Autodesk Fusion 360 part; units mm, degrees
(part 2 of 6)
  line L1135 (-27.0711, 10) -> (-22.9289, 10)
  line L1136 (-22.9289, 10) -> (-20, 12.9289)
  line L1137 (-20, 12.9289) -> (-20, 17.0711)
  line L1138 (-20, 17.0711) -> (-22.9289, 20)
  line L1139 (-20, 17.0711) -> (-20, 12.9289)
  line L1140 (-17.0711, 20) -> (-20, 17.0711)
  line L1141 (-16.6569, 19) -> (-19, 16.6569)
  line L1142 (-13.3431, 19) -> (-16.6569, 19)
  line L1143 (-11, 16.6569) -> (-13.3431, 19)
  line L1144 (-11, 13.3431) -> (-11, 16.6569)
  line L1145 (-13.3431, 11) -> (-11, 13.3431)
  line L1146 (-16.6569, 11) -> (-13.3431, 11)
  line L1147 (-19, 13.3431) -> (-16.6569, 11)
  line L1148 (-19, 16.6569) -> (-19, 13.3431)
  line L1149 (-20, 12.9289) -> (-17.0711, 10)
  line L1150 (-17.0711, 10) -> (-12.9289, 10)
  line L1151 (-12.9289, 10) -> (-10, 12.9289)
  line L1152 (-10, 12.9289) -> (-10, 17.0711)
  line L1153 (-10, 17.0711) -> (-12.9289, 20)
  line L1154 (-10, 17.0711) -> (-10, 12.9289)
  line L1155 (-7.0711, 20) -> (-10, 17.0711)
  line L1156 (-6.6569, 19) -> (-9, 16.6569)
  line L1157 (-3.3431, 19) -> (-6.6569, 19)
  line L1158 (-1, 16.6569) -> (-3.3431, 19)
  line L1159 (-1, 13.3431) -> (-1, 16.6569)
  line L1160 (-3.3431, 11) -> (-1, 13.3431)
  line L1161 (-6.6569, 11) -> (-3.3431, 11)
  line L1162 (-9, 13.3431) -> (-6.6569, 11)
  line L1163 (-9, 16.6569) -> (-9, 13.3431)
  line L1164 (-10, 12.9289) -> (-7.0711, 10)
  line L1165 (-7.0711, 10) -> (-2.9289, 10)
  line L1166 (-2.9289, 10) -> (0, 12.9289)
  line L1167 (0, 12.9289) -> (0, 17.0711)
  line L1168 (0, 17.0711) -> (-2.9289, 20)
  line L1169 (0, 17.0711) -> (0, 12.9289)
  line L1170 (2.9289, 20) -> (0, 17.0711)
  line L1171 (3.3431, 19) -> (1, 16.6569)
  line L1172 (6.6569, 19) -> (3.3431, 19)
  line L1173 (9, 16.6569) -> (6.6569, 19)
  line L1174 (9, 13.3431) -> (9, 16.6569)
  line L1175 (6.6569, 11) -> (9, 13.3431)
  line L1176 (3.3431, 11) -> (6.6569, 11)
  line L1177 (1, 13.3431) -> (3.3431, 11)
  line L1178 (1, 16.6569) -> (1, 13.3431)
  line L1179 (0, 12.9289) -> (2.9289, 10)
  line L1180 (2.9289, 10) -> (7.0711, 10)
  line L1181 (7.0711, 10) -> (10, 12.9289)
  line L1182 (10, 12.9289) -> (10, 17.0711)
  line L1183 (10, 17.0711) -> (7.0711, 20)
  line L1184 (10, 17.0711) -> (10, 12.9289)
  line L1185 (12.9289, 20) -> (10, 17.0711)
  line L1186 (13.3431, 19) -> (11, 16.6569)
  line L1187 (16.6569, 19) -> (13.3431, 19)
  line L1188 (19, 16.6569) -> (16.6569, 19)
  line L1189 (19, 13.3431) -> (19, 16.6569)
  line L1190 (16.6569, 11) -> (19, 13.3431)
  line L1191 (13.3431, 11) -> (16.6569, 11)
  line L1192 (11, 13.3431) -> (13.3431, 11)
  line L1193 (11, 16.6569) -> (11, 13.3431)
  line L1194 (10, 12.9289) -> (12.9289, 10)
  line L1195 (12.9289, 10) -> (17.0711, 10)
  line L1196 (17.0711, 10) -> (20, 12.9289)
  line L1197 (20, 12.9289) -> (20, 17.0711)
  line L1198 (20, 17.0711) -> (17.0711, 20)
  line L1199 (20, 17.0711) -> (20, 12.9289)
  line L1200 (22.9289, 20) -> (20, 17.0711)
  line L1201 (23.3431, 19) -> (21, 16.6569)
  line L1202 (26.6569, 19) -> (23.3431, 19)
  line L1203 (29, 16.6569) -> (26.6569, 19)
  line L1204 (29, 13.3431) -> (29, 16.6569)
  line L1205 (26.6569, 11) -> (29, 13.3431)
  line L1206 (23.3431, 11) -> (26.6569, 11)
  line L1207 (21, 13.3431) -> (23.3431, 11)
  line L1208 (21, 16.6569) -> (21, 13.3431)
  line L1209 (20, 12.9289) -> (22.9289, 10)
  line L1210 (22.9289, 10) -> (27.0711, 10)
  line L1211 (27.0711, 10) -> (30, 12.9289)
  line L1212 (30, 12.9289) -> (30, 17.0711)
  line L1213 (30, 17.0711) -> (27.0711, 20)
  line L1214 (30, 17.0711) -> (30, 12.9289)
  line L1215 (32.9289, 20) -> (30, 17.0711)
  line L1216 (33.3431, 19) -> (31, 16.6569)
  line L1217 (36.6569, 19) -> (33.3431, 19)
  line L1218 (39, 16.6569) -> (36.6569, 19)
  line L1219 (39, 13.3431) -> (39, 16.6569)
  line L1220 (36.6569, 11) -> (39, 13.3431)
  line L1221 (33.3431, 11) -> (36.6569, 11)
  line L1222 (31, 13.3431) -> (33.3431, 11)
  line L1223 (31, 16.6569) -> (31, 13.3431)
  line L1224 (30, 12.9289) -> (32.9289, 10)
  line L1225 (32.9289, 10) -> (37.0711, 10)
  line L1226 (37.0711, 10) -> (40, 12.9289)
  line L1227 (40, 12.9289) -> (40, 17.0711)
  line L1228 (40, 17.0711) -> (37.0711, 20)
  line L1229 (40, 17.0711) -> (40, 12.9289)
  line L1230 (42.9289, 20) -> (40, 17.0711)
  line L1231 (43.3431, 19) -> (41, 16.6569)
  line L1232 (46.6569, 19) -> (43.3431, 19)
  line L1233 (49, 16.6569) -> (46.6569, 19)
  line L1234 (49, 13.3431) -> (49, 16.6569)
  line L1235 (46.6569, 11) -> (49, 13.3431)
  line L1236 (43.3431, 11) -> (46.6569, 11)
  line L1237 (41, 13.3431) -> (43.3431, 11)
  line L1238 (41, 16.6569) -> (41, 13.3431)
  line L1239 (40, 12.9289) -> (42.9289, 10)
  line L1240 (42.9289, 10) -> (47.0711, 10)
  line L1241 (47.0711, 10) -> (50, 12.9289)
  line L1242 (50, 12.9289) -> (50, 17.0711)
  line L1243 (50, 17.0711) -> (47.0711, 20)
  line L1244 (50, 17.0711) -> (50, 12.9289)
  line L1245 (52.9289, 20) -> (50, 17.0711)
  line L1246 (53.3431, 19) -> (51, 16.6569)
  line L1247 (56.6569, 19) -> (53.3431, 19)
  line L1248 (59, 16.6569) -> (56.6569, 19)
  line L1249 (59, 13.3431) -> (59, 16.6569)
  line L1250 (56.6569, 11) -> (59, 13.3431)
  line L1251 (53.3431, 11) -> (56.6569, 11)
  line L1252 (51, 13.3431) -> (53.3431, 11)
  line L1253 (51, 16.6569) -> (51, 13.3431)
  line L1254 (50, 12.9289) -> (52.9289, 10)
  line L1255 (52.9289, 10) -> (57.0711, 10)
  line L1256 (57.0711, 10) -> (60, 12.9289)
  line L1257 (60, 12.9289) -> (60, 17.0711)
  line L1258 (60, 17.0711) -> (57.0711, 20)
  line L1259 (60, 17.0711) -> (60, 12.9289)
  line L1260 (62.9289, 20) -> (60, 17.0711)
  line L1261 (63.3431, 19) -> (61, 16.6569)
  line L1262 (66.6569, 19) -> (63.3431, 19)
  line L1263 (69, 16.6569) -> (66.6569, 19)
  line L1264 (69, 13.3431) -> (69, 16.6569)
  line L1265 (66.6569, 11) -> (69, 13.3431)
  line L1266 (63.3431, 11) -> (66.6569, 11)
  line L1267 (61, 13.3431) -> (63.3431, 11)
  line L1268 (61, 16.6569) -> (61, 13.3431)
  line L1269 (60, 12.9289) -> (62.9289, 10)
  line L1270 (62.9289, 10) -> (67.0711, 10)
  line L1271 (67.0711, 10) -> (70, 12.9289)
  line L1272 (70, 12.9289) -> (70, 17.0711)
  line L1273 (70, 17.0711) -> (67.0711, 20)
  line L1274 (-70, 7.0711) -> (-70, 2.9289)
  line L1275 (-67.0711, 10) -> (-70, 7.0711)
  line L1276 (-66.6569, 9) -> (-69, 6.6569)
  line L1277 (-63.3431, 9) -> (-66.6569, 9)
  line L1278 (-61, 6.6569) -> (-63.3431, 9)
  line L1279 (-61, 3.3431) -> (-61, 6.6569)
  line L1280 (-63.3431, 1) -> (-61, 3.3431)
  line L1281 (-66.6569, 1) -> (-63.3431, 1)
  line L1282 (-69, 3.3431) -> (-66.6569, 1)
  line L1283 (-69, 6.6569) -> (-69, 3.3431)
  line L1284 (-70, 2.9289) -> (-67.0711, 0)
  line L1285 (-67.0711, 0) -> (-62.9289, 0)
  line L1286 (-62.9289, 0) -> (-60, 2.9289)
  line L1287 (-60, 2.9289) -> (-60, 7.0711)
  line L1288 (-60, 7.0711) -> (-62.9289, 10)
  line L1289 (-60, 7.0711) -> (-60, 2.9289)
  line L1290 (-57.0711, 10) -> (-60, 7.0711)
  line L1291 (-56.6569, 9) -> (-59, 6.6569)
  line L1292 (-53.3431, 9) -> (-56.6569, 9)
  line L1293 (-51, 6.6569) -> (-53.3431, 9)
  line L1294 (-51, 3.3431) -> (-51, 6.6569)
  line L1295 (-53.3431, 1) -> (-51, 3.3431)
  line L1296 (-56.6569, 1) -> (-53.3431, 1)
  line L1297 (-59, 3.3431) -> (-56.6569, 1)
  line L1298 (-59, 6.6569) -> (-59, 3.3431)
  line L1299 (-60, 2.9289) -> (-57.0711, 0)
  line L1300 (-57.0711, 0) -> (-52.9289, 0)
  line L1301 (-52.9289, 0) -> (-50, 2.9289)
  line L1302 (-50, 2.9289) -> (-50, 7.0711)
  line L1303 (-50, 7.0711) -> (-52.9289, 10)
  line L1304 (-50, 7.0711) -> (-50, 2.9289)
  line L1305 (-47.0711, 10) -> (-50, 7.0711)
  line L1306 (-46.6569, 9) -> (-49, 6.6569)
  line L1307 (-43.3431, 9) -> (-46.6569, 9)
  line L1308 (-41, 6.6569) -> (-43.3431, 9)
  line L1309 (-41, 3.3431) -> (-41, 6.6569)
  line L1310 (-43.3431, 1) -> (-41, 3.3431)
  line L1311 (-46.6569, 1) -> (-43.3431, 1)
  line L1312 (-49, 3.3431) -> (-46.6569, 1)
  line L1313 (-49, 6.6569) -> (-49, 3.3431)
  line L1314 (-50, 2.9289) -> (-47.0711, 0)
  line L1315 (-47.0711, 0) -> (-42.9289, 0)
  line L1316 (-42.9289, 0) -> (-40, 2.9289)
  line L1317 (-40, 2.9289) -> (-40, 7.0711)
  line L1318 (-40, 7.0711) -> (-42.9289, 10)
  line L1319 (-40, 7.0711) -> (-40, 2.9289)
  line L1320 (-37.0711, 10) -> (-40, 7.0711)
  line L1321 (-36.6569, 9) -> (-39, 6.6569)
  line L1322 (-33.3431, 9) -> (-36.6569, 9)
  line L1323 (-31, 6.6569) -> (-33.3431, 9)
  line L1324 (-31, 3.3431) -> (-31, 6.6569)
  line L1325 (-33.3431, 1) -> (-31, 3.3431)
  line L1326 (-36.6569, 1) -> (-33.3431, 1)
  line L1327 (-39, 3.3431) -> (-36.6569, 1)
  line L1328 (-39, 6.6569) -> (-39, 3.3431)
  line L1329 (-40, 2.9289) -> (-37.0711, 0)
  line L1330 (-37.0711, 0) -> (-32.9289, 0)
  line L1331 (-32.9289, 0) -> (-30, 2.9289)
  line L1332 (-30, 2.9289) -> (-30, 7.0711)
  line L1333 (-30, 7.0711) -> (-32.9289, 10)
  line L1334 (-30, 7.0711) -> (-30, 2.9289)
  line L1335 (-27.0711, 10) -> (-30, 7.0711)
  line L1336 (-26.6569, 9) -> (-29, 6.6569)
  line L1337 (-23.3431, 9) -> (-26.6569, 9)
  line L1338 (-21, 6.6569) -> (-23.3431, 9)
  line L1339 (-21, 3.3431) -> (-21, 6.6569)
  line L1340 (-23.3431, 1) -> (-21, 3.3431)
  line L1341 (-26.6569, 1) -> (-23.3431, 1)
  line L1342 (-29, 3.3431) -> (-26.6569, 1)
  line L1343 (-29, 6.6569) -> (-29, 3.3431)
  line L1344 (-30, 2.9289) -> (-27.0711, 0)
  line L1345 (-27.0711, 0) -> (-22.9289, 0)
  line L1346 (-22.9289, 0) -> (-20, 2.9289)
  line L1347 (-20, 2.9289) -> (-20, 7.0711)
  line L1348 (-20, 7.0711) -> (-22.9289, 10)
  line L1349 (-20, 7.0711) -> (-20, 2.9289)
  line L1350 (-17.0711, 10) -> (-20, 7.0711)
  line L1351 (-16.6569, 9) -> (-19, 6.6569)
  line L1352 (-13.3431, 9) -> (-16.6569, 9)
  line L1353 (-11, 6.6569) -> (-13.3431, 9)
  line L1354 (-11, 3.3431) -> (-11, 6.6569)
  line L1355 (-13.3431, 1) -> (-11, 3.3431)
  line L1356 (-16.6569, 1) -> (-13.3431, 1)
  line L1357 (-19, 3.3431) -> (-16.6569, 1)
  line L1358 (-19, 6.6569) -> (-19, 3.3431)
  line L1359 (-20, 2.9289) -> (-17.0711, 0)
  line L1360 (-17.0711, 0) -> (-12.9289, 0)
  line L1361 (-12.9289, 0) -> (-10, 2.9289)
  line L1362 (-10, 2.9289) -> (-10, 7.0711)
  line L1363 (-10, 7.0711) -> (-12.9289, 10)
  line L1364 (-10, 7.0711) -> (-10, 2.9289)
  line L1365 (-7.0711, 10) -> (-10, 7.0711)
  line L1366 (-6.6569, 9) -> (-9, 6.6569)
  line L1367 (-3.3431, 9) -> (-6.6569, 9)
  line L1368 (-1, 6.6569) -> (-3.3431, 9)
  line L1369 (-1, 3.3431) -> (-1, 6.6569)
  line L1370 (-3.3431, 1) -> (-1, 3.3431)
  line L1371 (-6.6569, 1) -> (-3.3431, 1)
  line L1372 (-9, 3.3431) -> (-6.6569, 1)
  line L1373 (-9, 6.6569) -> (-9, 3.3431)
  line L1374 (-10, 2.9289) -> (-7.0711, 0)
  line L1375 (-7.0711, 0) -> (-2.9289, 0)
  line L1376 (-2.9289, 0) -> (0, 2.9289)
  line L1377 (0, 2.9289) -> (0, 7.0711)
  line L1378 (0, 7.0711) -> (-2.9289, 10)
  line L1379 (0, 7.0711) -> (0, 2.9289)
  line L1380 (2.9289, 10) -> (0, 7.0711)
  line L1381 (3.3431, 9) -> (1, 6.6569)
  line L1382 (6.6569, 9) -> (3.3431, 9)
  line L1383 (9, 6.6569) -> (6.6569, 9)
  line L1384 (9, 3.3431) -> (9, 6.6569)
  line L1385 (6.6569, 1) -> (9, 3.3431)
  line L1386 (3.3431, 1) -> (6.6569, 1)
  line L1387 (1, 3.3431) -> (3.3431, 1)
  line L1388 (1, 6.6569) -> (1, 3.3431)
  line L1389 (0, 2.9289) -> (2.9289, 0)
  line L1390 (2.9289, 0) -> (7.0711, 0)
  line L1391 (7.0711, 0) -> (10, 2.9289)
  line L1392 (10, 2.9289) -> (10, 7.0711)
  line L1393 (10, 7.0711) -> (7.0711, 10)
  line L1394 (10, 7.0711) -> (10, 2.9289)
  line L1395 (12.9289, 10) -> (10, 7.0711)
  line L1396 (13.3431, 9) -> (11, 6.6569)
  line L1397 (16.6569, 9) -> (13.3431, 9)
  line L1398 (19, 6.6569) -> (16.6569, 9)
  line L1399 (19, 3.3431) -> (19, 6.6569)
  line L1400 (16.6569, 1) -> (19, 3.3431)
  line L1401 (13.3431, 1) -> (16.6569, 1)
  line L1402 (11, 3.3431) -> (13.3431, 1)
  line L1403 (11, 6.6569) -> (11, 3.3431)
  line L1404 (10, 2.9289) -> (12.9289, 0)
  line L1405 (12.9289, 0) -> (17.0711, 0)
  line L1406 (17.0711, 0) -> (20, 2.9289)
  line L1407 (20, 2.9289) -> (20, 7.0711)
  line L1408 (20, 7.0711) -> (17.0711, 10)
  line L1409 (20, 7.0711) -> (20, 2.9289)
  line L1410 (22.9289, 10) -> (20, 7.0711)
  line L1411 (23.3431, 9) -> (21, 6.6569)
  line L1412 (26.6569, 9) -> (23.3431, 9)
  line L1413 (29, 6.6569) -> (26.6569, 9)
  line L1414 (29, 3.3431) -> (29, 6.6569)
  line L1415 (26.6569, 1) -> (29, 3.3431)
  line L1416 (23.3431, 1) -> (26.6569, 1)
  line L1417 (21, 3.3431) -> (23.3431, 1)
  line L1418 (21, 6.6569) -> (21, 3.3431)
  line L1419 (20, 2.9289) -> (22.9289, 0)
  line L1420 (22.9289, 0) -> (27.0711, 0)
  line L1421 (27.0711, 0) -> (30, 2.9289)
  line L1422 (30, 2.9289) -> (30, 7.0711)
  line L1423 (30, 7.0711) -> (27.0711, 10)
  line L1424 (30, 7.0711) -> (30, 2.9289)
  line L1425 (32.9289, 10) -> (30, 7.0711)
  line L1426 (33.3431, 9) -> (31, 6.6569)
  line L1427 (36.6569, 9) -> (33.3431, 9)
  line L1428 (39, 6.6569) -> (36.6569, 9)
  line L1429 (39, 3.3431) -> (39, 6.6569)
  line L1430 (36.6569, 1) -> (39, 3.3431)
  line L1431 (33.3431, 1) -> (36.6569, 1)
  line L1432 (31, 3.3431) -> (33.3431, 1)
  line L1433 (31, 6.6569) -> (31, 3.3431)
  line L1434 (30, 2.9289) -> (32.9289, 0)
  line L1435 (32.9289, 0) -> (37.0711, 0)
  line L1436 (37.0711, 0) -> (40, 2.9289)
  line L1437 (40, 2.9289) -> (40, 7.0711)
  line L1438 (40, 7.0711) -> (37.0711, 10)
  line L1439 (40, 7.0711) -> (40, 2.9289)
  line L1440 (42.9289, 10) -> (40, 7.0711)
  line L1441 (43.3431, 9) -> (41, 6.6569)
  line L1442 (46.6569, 9) -> (43.3431, 9)
  line L1443 (49, 6.6569) -> (46.6569, 9)
  line L1444 (49, 3.3431) -> (49, 6.6569)
  line L1445 (46.6569, 1) -> (49, 3.3431)
  line L1446 (43.3431, 1) -> (46.6569, 1)
  line L1447 (41, 3.3431) -> (43.3431, 1)
  line L1448 (41, 6.6569) -> (41, 3.3431)
  line L1449 (40, 2.9289) -> (42.9289, 0)
  line L1450 (42.9289, 0) -> (47.0711, 0)
  line L1451 (47.0711, 0) -> (50, 2.9289)
  line L1452 (50, 2.9289) -> (50, 7.0711)
  line L1453 (50, 7.0711) -> (47.0711, 10)
  line L1454 (50, 7.0711) -> (50, 2.9289)
  line L1455 (52.9289, 10) -> (50, 7.0711)
  line L1456 (53.3431, 9) -> (51, 6.6569)
  line L1457 (56.6569, 9) -> (53.3431, 9)
  line L1458 (59, 6.6569) -> (56.6569, 9)
  line L1459 (59, 3.3431) -> (59, 6.6569)
  line L1460 (56.6569, 1) -> (59, 3.3431)
  line L1461 (53.3431, 1) -> (56.6569, 1)
  line L1462 (51, 3.3431) -> (53.3431, 1)
  line L1463 (51, 6.6569) -> (51, 3.3431)
  line L1464 (50, 2.9289) -> (52.9289, 0)
  line L1465 (52.9289, 0) -> (57.0711, 0)
  line L1466 (57.0711, 0) -> (60, 2.9289)
  line L1467 (60, 2.9289) -> (60, 7.0711)
  line L1468 (60, 7.0711) -> (57.0711, 10)
  line L1469 (60, 7.0711) -> (60, 2.9289)
  line L1470 (62.9289, 10) -> (60, 7.0711)
  line L1471 (63.3431, 9) -> (61, 6.6569)
  line L1472 (66.6569, 9) -> (63.3431, 9)
  line L1473 (69, 6.6569) -> (66.6569, 9)
  line L1474 (69, 3.3431) -> (69, 6.6569)
  line L1475 (66.6569, 1) -> (69, 3.3431)
  line L1476 (63.3431, 1) -> (66.6569, 1)
  line L1477 (61, 3.3431) -> (63.3431, 1)
  line L1478 (61, 6.6569) -> (61, 3.3431)
  line L1479 (60, 2.9289) -> (62.9289, 0)
  line L1480 (62.9289, 0) -> (67.0711, 0)
  line L1481 (67.0711, 0) -> (70, 2.9289)
  line L1482 (70, 2.9289) -> (70, 7.0711)
  line L1483 (70, 7.0711) -> (67.0711, 10)
  line L1484 (-70, -2.9289) -> (-70, -7.0711)
  line L1485 (-67.0711, 0) -> (-70, -2.9289)
  line L1486 (-66.6569, -1) -> (-69, -3.3431)
  line L1487 (-63.3431, -1) -> (-66.6569, -1)
  line L1488 (-61, -3.3431) -> (-63.3431, -1)
  line L1489 (-61, -6.6569) -> (-61, -3.3431)
  line L1490 (-63.3431, -9) -> (-61, -6.6569)
  line L1491 (-66.6569, -9) -> (-63.3431, -9)
  line L1492 (-69, -6.6569) -> (-66.6569, -9)
  line L1493 (-69, -3.3431) -> (-69, -6.6569)
  line L1494 (-70, -7.0711) -> (-67.0711, -10)
  line L1495 (-67.0711, -10) -> (-62.9289, -10)
  line L1496 (-62.9289, -10) -> (-60, -7.0711)
  line L1497 (-60, -7.0711) -> (-60, -2.9289)
  line L1498 (-60, -2.9289) -> (-62.9289, 0)
  line L1499 (-60, -2.9289) -> (-60, -7.0711)
  line L1500 (-57.0711, 0) -> (-60, -2.9289)
  line L1501 (-56.6569, -1) -> (-59, -3.3431)
  line L1502 (-53.3431, -1) -> (-56.6569, -1)
  line L1503 (-51, -3.3431) -> (-53.3431, -1)
  line L1504 (-51, -6.6569) -> (-51, -3.3431)
  line L1505 (-53.3431, -9) -> (-51, -6.6569)
  line L1506 (-56.6569, -9) -> (-53.3431, -9)
  line L1507 (-59, -6.6569) -> (-56.6569, -9)
  line L1508 (-59, -3.3431) -> (-59, -6.6569)
  line L1509 (-60, -7.0711) -> (-57.0711, -10)
  line L1510 (-57.0711, -10) -> (-52.9289, -10)
  line L1511 (-52.9289, -10) -> (-50, -7.0711)
  line L1512 (-50, -7.0711) -> (-50, -2.9289)
  line L1513 (-50, -2.9289) -> (-52.9289, 0)
  line L1514 (-50, -2.9289) -> (-50, -7.0711)
  line L1515 (-47.0711, 0) -> (-50, -2.9289)
  line L1516 (-46.6569, -1) -> (-49, -3.3431)
  line L1517 (-43.3431, -1) -> (-46.6569, -1)
  line L1518 (-41, -3.3431) -> (-43.3431, -1)
  line L1519 (-41, -6.6569) -> (-41, -3.3431)
  line L1520 (-43.3431, -9) -> (-41, -6.6569)
  line L1521 (-46.6569, -9) -> (-43.3431, -9)
  line L1522 (-49, -6.6569) -> (-46.6569, -9)
  line L1523 (-49, -3.3431) -> (-49, -6.6569)
  line L1524 (-50, -7.0711) -> (-47.0711, -10)
  line L1525 (-47.0711, -10) -> (-42.9289, -10)
  line L1526 (-42.9289, -10) -> (-40, -7.0711)
  line L1527 (-40, -7.0711) -> (-40, -2.9289)
  line L1528 (-40, -2.9289) -> (-42.9289, 0)
  line L1529 (-40, -2.9289) -> (-40, -7.0711)
  line L1530 (-37.0711, 0) -> (-40, -2.9289)
  line L1531 (-36.6569, -1) -> (-39, -3.3431)
  line L1532 (-33.3431, -1) -> (-36.6569, -1)
  line L1533 (-31, -3.3431) -> (-33.3431, -1)
  line L1534 (-31, -6.6569) -> (-31, -3.3431)
  line L1535 (-33.3431, -9) -> (-31, -6.6569)
  line L1536 (-36.6569, -9) -> (-33.3431, -9)
  line L1537 (-39, -6.6569) -> (-36.6569, -9)
  line L1538 (-39, -3.3431) -> (-39, -6.6569)
  line L1539 (-40, -7.0711) -> (-37.0711, -10)
  line L1540 (-37.0711, -10) -> (-32.9289, -10)
  line L1541 (-32.9289, -10) -> (-30, -7.0711)
  line L1542 (-30, -7.0711) -> (-30, -2.9289)
  line L1543 (-30, -2.9289) -> (-32.9289, 0)
  line L1544 (-30, -2.9289) -> (-30, -7.0711)
  line L1545 (-27.0711, 0) -> (-30, -2.9289)
  line L1546 (-26.6569, -1) -> (-29, -3.3431)
  line L1547 (-23.3431, -1) -> (-26.6569, -1)
  line L1548 (-21, -3.3431) -> (-23.3431, -1)
  line L1549 (-21, -6.6569) -> (-21, -3.3431)
  line L1550 (-23.3431, -9) -> (-21, -6.6569)
  line L1551 (-26.6569, -9) -> (-23.3431, -9)
  line L1552 (-29, -6.6569) -> (-26.6569, -9)
  line L1553 (-29, -3.3431) -> (-29, -6.6569)
  line L1554 (-30, -7.0711) -> (-27.0711, -10)
  line L1555 (-27.0711, -10) -> (-22.9289, -10)
  line L1556 (-22.9289, -10) -> (-20, -7.0711)
  line L1557 (-20, -7.0711) -> (-20, -2.9289)
  line L1558 (-20, -2.9289) -> (-22.9289, 0)
  line L1559 (-20, -2.9289) -> (-20, -7.0711)
  line L1560 (-17.0711, 0) -> (-20, -2.9289)
  line L1561 (-16.6569, -1) -> (-19, -3.3431)
  line L1562 (-13.3431, -1) -> (-16.6569, -1)
  line L1563 (-11, -3.3431) -> (-13.3431, -1)
  line L1564 (-11, -6.6569) -> (-11, -3.3431)
  line L1565 (-13.3431, -9) -> (-11, -6.6569)
  line L1566 (-16.6569, -9) -> (-13.3431, -9)
  line L1567 (-19, -6.6569) -> (-16.6569, -9)
  line L1568 (-19, -3.3431) -> (-19, -6.6569)
  line L1569 (-20, -7.0711) -> (-17.0711, -10)
  line L1570 (-17.0711, -10) -> (-12.9289, -10)
  line L1571 (-12.9289, -10) -> (-10, -7.0711)
  line L1572 (-10, -7.0711) -> (-10, -2.9289)
  line L1573 (-10, -2.9289) -> (-12.9289, 0)
  line L1574 (-10, -2.9289) -> (-10, -7.0711)
  line L1575 (-7.0711, 0) -> (-10, -2.9289)
  line L1576 (-6.6569, -1) -> (-9, -3.3431)
  line L1577 (-3.3431, -1) -> (-6.6569, -1)
  line L1578 (-1, -3.3431) -> (-3.3431, -1)
  line L1579 (-1, -6.6569) -> (-1, -3.3431)
  line L1580 (-3.3431, -9) -> (-1, -6.6569)
  line L1581 (-6.6569, -9) -> (-3.3431, -9)
  line L1582 (-9, -6.6569) -> (-6.6569, -9)
  line L1583 (-9, -3.3431) -> (-9, -6.6569)
  line L1584 (-10, -7.0711) -> (-7.0711, -10)
  line L1585 (-7.0711, -10) -> (-2.9289, -10)
  line L1586 (-2.9289, -10) -> (0, -7.0711)
  line L1587 (0, -7.0711) -> (0, -2.9289)
  line L1588 (0, -2.9289) -> (-2.9289, 0)
  line L1589 (0, -2.9289) -> (0, -7.0711)
  line L1590 (2.9289, 0) -> (0, -2.9289)
  line L1591 (3.3431, -1) -> (1, -3.3431)
  line L1592 (6.6569, -1) -> (3.3431, -1)
  line L1593 (9, -3.3431) -> (6.6569, -1)
  line L1594 (9, -6.6569) -> (9, -3.3431)
  line L1595 (6.6569, -9) -> (9, -6.6569)
  line L1596 (3.3431, -9) -> (6.6569, -9)
  line L1597 (1, -6.6569) -> (3.3431, -9)
  line L1598 (1, -3.3431) -> (1, -6.6569)
  line L1599 (0, -7.0711) -> (2.9289, -10)
  line L1600 (2.9289, -10) -> (7.0711, -10)
  line L1601 (7.0711, -10) -> (10, -7.0711)
  line L1602 (10, -7.0711) -> (10, -2.9289)
  line L1603 (10, -2.9289) -> (7.0711, 0)
  line L1604 (10, -2.9289) -> (10, -7.0711)
  line L1605 (12.9289, 0) -> (10, -2.9289)
  line L1606 (13.3431, -1) -> (11, -3.3431)
  line L1607 (16.6569, -1) -> (13.3431, -1)
  line L1608 (19, -3.3431) -> (16.6569, -1)
  line L1609 (19, -6.6569) -> (19, -3.3431)
  line L1610 (16.6569, -9) -> (19, -6.6569)
  line L1611 (13.3431, -9) -> (16.6569, -9)
  line L1612 (11, -6.6569) -> (13.3431, -9)
  line L1613 (11, -3.3431) -> (11, -6.6569)
  line L1614 (10, -7.0711) -> (12.9289, -10)
  line L1615 (12.9289, -10) -> (17.0711, -10)
  line L1616 (17.0711, -10) -> (20, -7.0711)
  line L1617 (20, -7.0711) -> (20, -2.9289)
  line L1618 (20, -2.9289) -> (17.0711, 0)
  line L1619 (20, -2.9289) -> (20, -7.0711)
  line L1620 (22.9289, 0) -> (20, -2.9289)
  line L1621 (23.3431, -1) -> (21, -3.3431)
  line L1622 (26.6569, -1) -> (23.3431, -1)
  line L1623 (29, -3.3431) -> (26.6569, -1)
  line L1624 (29, -6.6569) -> (29, -3.3431)
  line L1625 (26.6569, -9) -> (29, -6.6569)
  line L1626 (23.3431, -9) -> (26.6569, -9)
  line L1627 (21, -6.6569) -> (23.3431, -9)
  line L1628 (21, -3.3431) -> (21, -6.6569)
  line L1629 (20, -7.0711) -> (22.9289, -10)
  line L1630 (22.9289, -10) -> (27.0711, -10)
  line L1631 (27.0711, -10) -> (30, -7.0711)
  line L1632 (30, -7.0711) -> (30, -2.9289)
  line L1633 (30, -2.9289) -> (27.0711, 0)
  line L1634 (30, -2.9289) -> (30, -7.0711)
  line L1635 (32.9289, 0) -> (30, -2.9289)
  line L1636 (33.3431, -1) -> (31, -3.3431)
  line L1637 (36.6569, -1) -> (33.3431, -1)
  line L1638 (39, -3.3431) -> (36.6569, -1)
  line L1639 (39, -6.6569) -> (39, -3.3431)
  line L1640 (36.6569, -9) -> (39, -6.6569)
  line L1641 (33.3431, -9) -> (36.6569, -9)
  line L1642 (31, -6.6569) -> (33.3431, -9)
  line L1643 (31, -3.3431) -> (31, -6.6569)
  line L1644 (30, -7.0711) -> (32.9289, -10)
  line L1645 (32.9289, -10) -> (37.0711, -10)
  line L1646 (37.0711, -10) -> (40, -7.0711)
  line L1647 (40, -7.0711) -> (40, -2.9289)
  line L1648 (40, -2.9289) -> (37.0711, 0)
  line L1649 (40, -2.9289) -> (40, -7.0711)
  line L1650 (42.9289, 0) -> (40, -2.9289)
  line L1651 (43.3431, -1) -> (41, -3.3431)
  line L1652 (46.6569, -1) -> (43.3431, -1)
  line L1653 (49, -3.3431) -> (46.6569, -1)
  line L1654 (49, -6.6569) -> (49, -3.3431)
  line L1655 (46.6569, -9) -> (49, -6.6569)
  line L1656 (43.3431, -9) -> (46.6569, -9)
  line L1657 (41, -6.6569) -> (43.3431, -9)
  line L1658 (41, -3.3431) -> (41, -6.6569)
  line L1659 (40, -7.0711) -> (42.9289, -10)
  line L1660 (42.9289, -10) -> (47.0711, -10)
  line L1661 (47.0711, -10) -> (50, -7.0711)
  line L1662 (50, -7.0711) -> (50, -2.9289)
  line L1663 (50, -2.9289) -> (47.0711, 0)
  line L1664 (50, -2.9289) -> (50, -7.0711)
  line L1665 (52.9289, 0) -> (50, -2.9289)
  line L1666 (53.3431, -1) -> (51, -3.3431)
  line L1667 (56.6569, -1) -> (53.3431, -1)
  line L1668 (59, -3.3431) -> (56.6569, -1)
  line L1669 (59, -6.6569) -> (59, -3.3431)
  line L1670 (56.6569, -9) -> (59, -6.6569)
  line L1671 (53.3431, -9) -> (56.6569, -9)
  line L1672 (51, -6.6569) -> (53.3431, -9)
  line L1673 (51, -3.3431) -> (51, -6.6569)
  line L1674 (50, -7.0711) -> (52.9289, -10)
  line L1675 (52.9289, -10) -> (57.0711, -10)
  line L1676 (57.0711, -10) -> (60, -7.0711)
  line L1677 (60, -7.0711) -> (60, -2.9289)
  line L1678 (60, -2.9289) -> (57.0711, 0)
  line L1679 (60, -2.9289) -> (60, -7.0711)
  line L1680 (62.9289, 0) -> (60, -2.9289)
  line L1681 (63.3431, -1) -> (61, -3.3431)
  line L1682 (66.6569, -1) -> (63.3431, -1)
  line L1683 (69, -3.3431) -> (66.6569, -1)
  line L1684 (69, -6.6569) -> (69, -3.3431)
  line L1685 (66.6569, -9) -> (69, -6.6569)
  line L1686 (63.3431, -9) -> (66.6569, -9)
  line L1687 (61, -6.6569) -> (63.3431, -9)
  line L1688 (61, -3.3431) -> (61, -6.6569)
  line L1689 (60, -7.0711) -> (62.9289, -10)
  line L1690 (62.9289, -10) -> (67.0711, -10)
  line L1691 (67.0711, -10) -> (70, -7.0711)
  line L1692 (70, -7.0711) -> (70, -2.9289)
  line L1693 (70, -2.9289) -> (67.0711, 0)
  line L1694 (-70, -12.9289) -> (-70, -17.0711)
  line L1695 (-67.0711, -10) -> (-70, -12.9289)
  line L1696 (-66.6569, -11) -> (-69, -13.3431)
  line L1697 (-63.3431, -11) -> (-66.6569, -11)
  line L1698 (-61, -13.3431) -> (-63.3431, -11)
  line L1699 (-61, -16.6569) -> (-61, -13.3431)
  line L1700 (-63.3431, -19) -> (-61, -16.6569)
  line L1701 (-66.6569, -19) -> (-63.3431, -19)
  line L1702 (-69, -16.6569) -> (-66.6569, -19)
  line L1703 (-69, -13.3431) -> (-69, -16.6569)
  line L1704 (-70, -17.0711) -> (-67.0711, -20)
  line L1705 (-67.0711, -20) -> (-62.9289, -20)
  line L1706 (-62.9289, -20) -> (-60, -17.0711)
  line L1707 (-60, -17.0711) -> (-60, -12.9289)
  line L1708 (-60, -12.9289) -> (-62.9289, -10)
  line L1709 (-60, -12.9289) -> (-60, -17.0711)
  line L1710 (-57.0711, -10) -> (-60, -12.9289)
  line L1711 (-56.6569, -11) -> (-59, -13.3431)
  line L1712 (-53.3431, -11) -> (-56.6569, -11)
  line L1713 (-51, -13.3431) -> (-53.3431, -11)
  line L1714 (-51, -16.6569) -> (-51, -13.3431)
  line L1715 (-53.3431, -19) -> (-51, -16.6569)
  line L1716 (-56.6569, -19) -> (-53.3431, -19)
  line L1717 (-59, -16.6569) -> (-56.6569, -19)
  line L1718 (-59, -13.3431) -> (-59, -16.6569)
  line L1719 (-60, -17.0711) -> (-57.0711, -20)
  line L1720 (-57.0711, -20) -> (-52.9289, -20)
  line L1721 (-52.9289, -20) -> (-50, -17.0711)
  line L1722 (-50, -17.0711) -> (-50, -12.9289)
  line L1723 (-50, -12.9289) -> (-52.9289, -10)
  line L1724 (-50, -12.9289) -> (-50, -17.0711)
  line L1725 (-47.0711, -10) -> (-50, -12.9289)
  line L1726 (-46.6569, -11) -> (-49, -13.3431)
  line L1727 (-43.3431, -11) -> (-46.6569, -11)
  line L1728 (-41, -13.3431) -> (-43.3431, -11)
  line L1729 (-41, -16.6569) -> (-41, -13.3431)
  line L1730 (-43.3431, -19) -> (-41, -16.6569)
  line L1731 (-46.6569, -19) -> (-43.3431, -19)
  line L1732 (-49, -16.6569) -> (-46.6569, -19)
  line L1733 (-49, -13.3431) -> (-49, -16.6569)
  line L1734 (-50, -17.0711) -> (-47.0711, -20)
  line L1735 (-47.0711, -20) -> (-42.9289, -20)
  line L1736 (-42.9289, -20) -> (-40, -17.0711)
  line L1737 (-40, -17.0711) -> (-40, -12.9289)
  line L1738 (-40, -12.9289) -> (-42.9289, -10)
  line L1739 (-40, -12.9289) -> (-40, -17.0711)
  line L1740 (-37.0711, -10) -> (-40, -12.9289)
  line L1741 (-36.6569, -11) -> (-39, -13.3431)
  line L1742 (-33.3431, -11) -> (-36.6569, -11)
  line L1743 (-31, -13.3431) -> (-33.3431, -11)
  line L1744 (-31, -16.6569) -> (-31, -13.3431)
  line L1745 (-33.3431, -19) -> (-31, -16.6569)
  line L1746 (-36.6569, -19) -> (-33.3431, -19)
  line L1747 (-39, -16.6569) -> (-36.6569, -19)
  line L1748 (-39, -13.3431) -> (-39, -16.6569)
  line L1749 (-40, -17.0711) -> (-37.0711, -20)
  line L1750 (-37.0711, -20) -> (-32.9289, -20)
  line L1751 (-32.9289, -20) -> (-30, -17.0711)
  line L1752 (-30, -17.0711) -> (-30, -12.9289)
  line L1753 (-30, -12.9289) -> (-32.9289, -10)
  line L1754 (-30, -12.9289) -> (-30, -17.0711)
  line L1755 (-27.0711, -10) -> (-30, -12.9289)
  line L1756 (-26.6569, -11) -> (-29, -13.3431)
  line L1757 (-23.3431, -11) -> (-26.6569, -11)
  line L1758 (-21, -13.3431) -> (-23.3431, -11)
  line L1759 (-21, -16.6569) -> (-21, -13.3431)
  line L1760 (-23.3431, -19) -> (-21, -16.6569)
  line L1761 (-26.6569, -19) -> (-23.3431, -19)
  line L1762 (-29, -16.6569) -> (-26.6569, -19)
  line L1763 (-29, -13.3431) -> (-29, -16.6569)
  line L1764 (-30, -17.0711) -> (-27.0711, -20)
  line L1765 (-27.0711, -20) -> (-22.9289, -20)
  line L1766 (-22.9289, -20) -> (-20, -17.0711)
  line L1767 (-20, -17.0711) -> (-20, -12.9289)
  line L1768 (-20, -12.9289) -> (-22.9289, -10)
  line L1769 (-20, -12.9289) -> (-20, -17.0711)
  line L1770 (-17.0711, -10) -> (-20, -12.9289)
  line L1771 (-16.6569, -11) -> (-19, -13.3431)
  line L1772 (-13.3431, -11) -> (-16.6569, -11)
  line L1773 (-11, -13.3431) -> (-13.3431, -11)
  line L1774 (-11, -16.6569) -> (-11, -13.3431)
  line L1775 (-13.3431, -19) -> (-11, -16.6569)
  line L1776 (-16.6569, -19) -> (-13.3431, -19)
  line L1777 (-19, -16.6569) -> (-16.6569, -19)
  line L1778 (-19, -13.3431) -> (-19, -16.6569)
  line L1779 (-20, -17.0711) -> (-17.0711, -20)
  line L1780 (-17.0711, -20) -> (-12.9289, -20)
  line L1781 (-12.9289, -20) -> (-10, -17.0711)
  line L1782 (-10, -17.0711) -> (-10, -12.9289)
  line L1783 (-10, -12.9289) -> (-12.9289, -10)
  line L1784 (-10, -12.9289) -> (-10, -17.0711)
  line L1785 (-7.0711, -10) -> (-10, -12.9289)
  line L1786 (-6.6569, -11) -> (-9, -13.3431)
  line L1787 (-3.3431, -11) -> (-6.6569, -11)
  line L1788 (-1, -13.3431) -> (-3.3431, -11)
  line L1789 (-1, -16.6569) -> (-1, -13.3431)
  line L1790 (-3.3431, -19) -> (-1, -16.6569)
  line L1791 (-6.6569, -19) -> (-3.3431, -19)
  line L1792 (-9, -16.6569) -> (-6.6569, -19)
  line L1793 (-9, -13.3431) -> (-9, -16.6569)
  line L1794 (-10, -17.0711) -> (-7.0711, -20)
  line L1795 (-7.0711, -20) -> (-2.9289, -20)
  line L1796 (-2.9289, -20) -> (0, -17.0711)
  line L1797 (0, -17.0711) -> (0, -12.9289)
  line L1798 (0, -12.9289) -> (-2.9289, -10)
  line L1799 (0, -12.9289) -> (0, -17.0711)
  line L1800 (2.9289, -10) -> (0, -12.9289)
  line L1801 (3.3431, -11) -> (1, -13.3431)
  line L1802 (6.6569, -11) -> (3.3431, -11)
  line L1803 (9, -13.3431) -> (6.6569, -11)
  line L1804 (9, -16.6569) -> (9, -13.3431)
  line L1805 (6.6569, -19) -> (9, -16.6569)
  line L1806 (3.3431, -19) -> (6.6569, -19)
  line L1807 (1, -16.6569) -> (3.3431, -19)
  line L1808 (1, -13.3431) -> (1, -16.6569)
  line L1809 (0, -17.0711) -> (2.9289, -20)
  line L1810 (2.9289, -20) -> (7.0711, -20)
  line L1811 (7.0711, -20) -> (10, -17.0711)
  line L1812 (10, -17.0711) -> (10, -12.9289)
  line L1813 (10, -12.9289) -> (7.0711, -10)
  line L1814 (10, -12.9289) -> (10, -17.0711)
  line L1815 (12.9289, -10) -> (10, -12.9289)
  line L1816 (13.3431, -11) -> (11, -13.3431)
  line L1817 (16.6569, -11) -> (13.3431, -11)
  line L1818 (19, -13.3431) -> (16.6569, -11)
  line L1819 (19, -16.6569) -> (19, -13.3431)
  line L1820 (16.6569, -19) -> (19, -16.6569)
  line L1821 (13.3431, -19) -> (16.6569, -19)
  line L1822 (11, -16.6569) -> (13.3431, -19)
  line L1823 (11, -13.3431) -> (11, -16.6569)
  line L1824 (10, -17.0711) -> (12.9289, -20)
  line L1825 (12.9289, -20) -> (17.0711, -20)
  line L1826 (17.0711, -20) -> (20, -17.0711)
  line L1827 (20, -17.0711) -> (20, -12.9289)
  line L1828 (20, -12.9289) -> (17.0711, -10)
  line L1829 (20, -12.9289) -> (20, -17.0711)
  line L1830 (22.9289, -10) -> (20, -12.9289)
  line L1831 (23.3431, -11) -> (21, -13.3431)
  line L1832 (26.6569, -11) -> (23.3431, -11)
  line L1833 (29, -13.3431) -> (26.6569, -11)
  line L1834 (29, -16.6569) -> (29, -13.3431)
  line L1835 (26.6569, -19) -> (29, -16.6569)
  line L1836 (23.3431, -19) -> (26.6569, -19)
  line L1837 (21, -16.6569) -> (23.3431, -19)
  line L1838 (21, -13.3431) -> (21, -16.6569)
  line L1839 (20, -17.0711) -> (22.9289, -20)
  line L1840 (22.9289, -20) -> (27.0711, -20)
  line L1841 (27.0711, -20) -> (30, -17.0711)
  line L1842 (30, -17.0711) -> (30, -12.9289)
  line L1843 (30, -12.9289) -> (27.0711, -10)
  line L1844 (30, -12.9289) -> (30, -17.0711)
  line L1845 (32.9289, -10) -> (30, -12.9289)
  line L1846 (33.3431, -11) -> (31, -13.3431)
  line L1847 (36.6569, -11) -> (33.3431, -11)
  line L1848 (39, -13.3431) -> (36.6569, -11)
  line L1849 (39, -16.6569) -> (39, -13.3431)
  line L1850 (36.6569, -19) -> (39, -16.6569)
  line L1851 (33.3431, -19) -> (36.6569, -19)
  line L1852 (31, -16.6569) -> (33.3431, -19)
  line L1853 (31, -13.3431) -> (31, -16.6569)
  line L1854 (30, -17.0711) -> (32.9289, -20)
  line L1855 (32.9289, -20) -> (37.0711, -20)
  line L1856 (37.0711, -20) -> (40, -17.0711)
  line L1857 (40, -17.0711) -> (40, -12.9289)
  line L1858 (40, -12.9289) -> (37.0711, -10)
  line L1859 (40, -12.9289) -> (40, -17.0711)
  line L1860 (42.9289, -10) -> (40, -12.9289)
  line L1861 (43.3431, -11) -> (41, -13.3431)
  line L1862 (46.6569, -11) -> (43.3431, -11)
  line L1863 (49, -13.3431) -> (46.6569, -11)
  line L1864 (49, -16.6569) -> (49, -13.3431)
  line L1865 (46.6569, -19) -> (49, -16.6569)
  line L1866 (43.3431, -19) -> (46.6569, -19)
  line L1867 (41, -16.6569) -> (43.3431, -19)
  line L1868 (41, -13.3431) -> (41, -16.6569)
  line L1869 (40, -17.0711) -> (42.9289, -20)
  line L1870 (42.9289, -20) -> (47.0711, -20)
  line L1871 (47.0711, -20) -> (50, -17.0711)
  line L1872 (50, -17.0711) -> (50, -12.9289)
  line L1873 (50, -12.9289) -> (47.0711, -10)
  line L1874 (50, -12.9289) -> (50, -17.0711)
  line L1875 (52.9289, -10) -> (50, -12.9289)
  line L1876 (53.3431, -11) -> (51, -13.3431)
  line L1877 (56.6569, -11) -> (53.3431, -11)
  line L1878 (59, -13.3431) -> (56.6569, -11)
  line L1879 (59, -16.6569) -> (59, -13.3431)
  line L1880 (56.6569, -19) -> (59, -16.6569)
  line L1881 (53.3431, -19) -> (56.6569, -19)
  line L1882 (51, -16.6569) -> (53.3431, -19)
  line L1883 (51, -13.3431) -> (51, -16.6569)
  line L1884 (50, -17.0711) -> (52.9289, -20)
  line L1885 (52.9289, -20) -> (57.0711, -20)
  line L1886 (57.0711, -20) -> (60, -17.0711)
  line L1887 (60, -17.0711) -> (60, -12.9289)
  line L1888 (60, -12.9289) -> (57.0711, -10)
  line L1889 (60, -12.9289) -> (60, -17.0711)
  line L1890 (62.9289, -10) -> (60, -12.9289)
  line L1891 (63.3431, -11) -> (61, -13.3431)
  line L1892 (66.6569, -11) -> (63.3431, -11)
  line L1893 (69, -13.3431) -> (66.6569, -11)
  line L1894 (69, -16.6569) -> (69, -13.3431)
  line L1895 (66.6569, -19) -> (69, -16.6569)
  line L1896 (63.3431, -19) -> (66.6569, -19)
  line L1897 (61, -16.6569) -> (63.3431, -19)
  line L1898 (61, -13.3431) -> (61, -16.6569)
  line L1899 (60, -17.0711) -> (62.9289, -20)
  line L1900 (62.9289, -20) -> (67.0711, -20)
  line L1901 (67.0711, -20) -> (70, -17.0711)
  line L1902 (70, -17.0711) -> (70, -12.9289)
  line L1903 (70, -12.9289) -> (67.0711, -10)
  line L1904 (-70, -22.9289) -> (-70, -27.0711)
  line L1905 (-67.0711, -20) -> (-70, -22.9289)
  line L1906 (-66.6569, -21) -> (-69, -23.3431)
  line L1907 (-63.3431, -21) -> (-66.6569, -21)
  line L1908 (-61, -23.3431) -> (-63.3431, -21)
  line L1909 (-61, -26.6569) -> (-61, -23.3431)
  line L1910 (-63.3431, -29) -> (-61, -26.6569)
  line L1911 (-66.6569, -29) -> (-63.3431, -29)
  line L1912 (-69, -26.6569) -> (-66.6569, -29)
  line L1913 (-69, -23.3431) -> (-69, -26.6569)
  line L1914 (-70, -27.0711) -> (-67.0711, -30)
  line L1915 (-67.0711, -30) -> (-62.9289, -30)
  line L1916 (-62.9289, -30) -> (-60, -27.0711)
  line L1917 (-60, -27.0711) -> (-60, -22.9289)
  line L1918 (-60, -22.9289) -> (-62.9289, -20)
  line L1919 (-60, -22.9289) -> (-60, -27.0711)
  line L1920 (-57.0711, -20) -> (-60, -22.9289)
  line L1921 (-56.6569, -21) -> (-59, -23.3431)
  line L1922 (-53.3431, -21) -> (-56.6569, -21)
  line L1923 (-51, -23.3431) -> (-53.3431, -21)
  line L1924 (-51, -26.6569) -> (-51, -23.3431)
  line L1925 (-53.3431, -29) -> (-51, -26.6569)
  line L1926 (-56.6569, -29) -> (-53.3431, -29)
  line L1927 (-59, -26.6569) -> (-56.6569, -29)
  line L1928 (-59, -23.3431) -> (-59, -26.6569)
  line L1929 (-60, -27.0711) -> (-57.0711, -30)
  line L1930 (-57.0711, -30) -> (-52.9289, -30)
  line L1931 (-52.9289, -30) -> (-50, -27.0711)
  line L1932 (-50, -27.0711) -> (-50, -22.9289)
  line L1933 (-50, -22.9289) -> (-52.9289, -20)
  line L1934 (-50, -22.9289) -> (-50, -27.0711)
  line L1935 (-47.0711, -20) -> (-50, -22.9289)
  line L1936 (-46.6569, -21) -> (-49, -23.3431)
  line L1937 (-43.3431, -21) -> (-46.6569, -21)
  line L1938 (-41, -23.3431) -> (-43.3431, -21)
  line L1939 (-41, -26.6569) -> (-41, -23.3431)
  line L1940 (-43.3431, -29) -> (-41, -26.6569)
  line L1941 (-46.6569, -29) -> (-43.3431, -29)
  line L1942 (-49, -26.6569) -> (-46.6569, -29)
  line L1943 (-49, -23.3431) -> (-49, -26.6569)
  line L1944 (-50, -27.0711) -> (-47.0711, -30)
  line L1945 (-47.0711, -30) -> (-42.9289, -30)
  line L1946 (-42.9289, -30) -> (-40, -27.0711)
  line L1947 (-40, -27.0711) -> (-40, -22.9289)
  line L1948 (-40, -22.9289) -> (-42.9289, -20)
  line L1949 (-40, -22.9289) -> (-40, -27.0711)
  line L1950 (-37.0711, -20) -> (-40, -22.9289)
  line L1951 (-36.6569, -21) -> (-39, -23.3431)
  line L1952 (-33.3431, -21) -> (-36.6569, -21)
  line L1953 (-31, -23.3431) -> (-33.3431, -21)
  line L1954 (-31, -26.6569) -> (-31, -23.3431)
  line L1955 (-33.3431, -29) -> (-31, -26.6569)
  line L1956 (-36.6569, -29) -> (-33.3431, -29)
  line L1957 (-39, -26.6569) -> (-36.6569, -29)
  line L1958 (-39, -23.3431) -> (-39, -26.6569)
  line L1959 (-40, -27.0711) -> (-37.0711, -30)
  line L1960 (-37.0711, -30) -> (-32.9289, -30)
  line L1961 (-32.9289, -30) -> (-30, -27.0711)
  line L1962 (-30, -27.0711) -> (-30, -22.9289)
  line L1963 (-30, -22.9289) -> (-32.9289, -20)
  line L1964 (-30, -22.9289) -> (-30, -27.0711)
  line L1965 (-27.0711, -20) -> (-30, -22.9289)
  line L1966 (-26.6569, -21) -> (-29, -23.3431)
  line L1967 (-23.3431, -21) -> (-26.6569, -21)
  line L1968 (-21, -23.3431) -> (-23.3431, -21)
  line L1969 (-21, -26.6569) -> (-21, -23.3431)
  line L1970 (-23.3431, -29) -> (-21, -26.6569)
  line L1971 (-26.6569, -29) -> (-23.3431, -29)
  line L1972 (-29, -26.6569) -> (-26.6569, -29)
  line L1973 (-29, -23.3431) -> (-29, -26.6569)
  line L1974 (-30, -27.0711) -> (-27.0711, -30)
  line L1975 (-27.0711, -30) -> (-22.9289, -30)
  line L1976 (-22.9289, -30) -> (-20, -27.0711)
  line L1977 (-20, -27.0711) -> (-20, -22.9289)
  line L1978 (-20, -22.9289) -> (-22.9289, -20)
  line L1979 (-20, -22.9289) -> (-20, -27.0711)
  line L1980 (-17.0711, -20) -> (-20, -22.9289)
  line L1981 (-16.6569, -21) -> (-19, -23.3431)
  line L1982 (-13.3431, -21) -> (-16.6569, -21)
  line L1983 (-11, -23.3431) -> (-13.3431, -21)
  line L1984 (-11, -26.6569) -> (-11, -23.3431)
  line L1985 (-13.3431, -29) -> (-11, -26.6569)
  line L1986 (-16.6569, -29) -> (-13.3431, -29)
  line L1987 (-19, -26.6569) -> (-16.6569, -29)
  line L1988 (-19, -23.3431) -> (-19, -26.6569)
  line L1989 (-20, -27.0711) -> (-17.0711, -30)
  line L1990 (-17.0711, -30) -> (-12.9289, -30)
  line L1991 (-12.9289, -30) -> (-10, -27.0711)
  line L1992 (-10, -27.0711) -> (-10, -22.9289)
  line L1993 (-10, -22.9289) -> (-12.9289, -20)
  line L1994 (-10, -22.9289) -> (-10, -27.0711)
  line L1995 (-7.0711, -20) -> (-10, -22.9289)
  line L1996 (-6.6569, -21) -> (-9, -23.3431)
  line L1997 (-3.3431, -21) -> (-6.6569, -21)
  line L1998 (-1, -23.3431) -> (-3.3431, -21)
  line L1999 (-1, -26.6569) -> (-1, -23.3431)
  line L2000 (-3.3431, -29) -> (-1, -26.6569)
  line L2001 (-6.6569, -29) -> (-3.3431, -29)
  line L2002 (-9, -26.6569) -> (-6.6569, -29)
  line L2003 (-9, -23.3431) -> (-9, -26.6569)
  line L2004 (-10, -27.0711) -> (-7.0711, -30)
  line L2005 (-7.0711, -30) -> (-2.9289, -30)
  line L2006 (-2.9289, -30) -> (0, -27.0711)
  line L2007 (0, -27.0711) -> (0, -22.9289)
  line L2008 (0, -22.9289) -> (-2.9289, -20)
  line L2009 (0, -22.9289) -> (0, -27.0711)
  line L2010 (2.9289, -20) -> (0, -22.9289)
  line L2011 (3.3431, -21) -> (1, -23.3431)
  line L2012 (6.6569, -21) -> (3.3431, -21)
  line L2013 (9, -23.3431) -> (6.6569, -21)
  line L2014 (9, -26.6569) -> (9, -23.3431)
  line L2015 (6.6569, -29) -> (9, -26.6569)
  line L2016 (3.3431, -29) -> (6.6569, -29)
  line L2017 (1, -26.6569) -> (3.3431, -29)
  line L2018 (1, -23.3431) -> (1, -26.6569)
  line L2019 (0, -27.0711) -> (2.9289, -30)
  line L2020 (2.9289, -30) -> (7.0711, -30)
  line L2021 (7.0711, -30) -> (10, -27.0711)
  line L2022 (10, -27.0711) -> (10, -22.9289)
  line L2023 (10, -22.9289) -> (7.0711, -20)
  line L2024 (10, -22.9289) -> (10, -27.0711)
  line L2025 (12.9289, -20) -> (10, -22.9289)
  line L2026 (13.3431, -21) -> (11, -23.3431)
  line L2027 (16.6569, -21) -> (13.3431, -21)
  line L2028 (19, -23.3431) -> (16.6569, -21)
  line L2029 (19, -26.6569) -> (19, -23.3431)
  line L2030 (16.6569, -29) -> (19, -26.6569)
  line L2031 (13.3431, -29) -> (16.6569, -29)
  line L2032 (11, -26.6569) -> (13.3431, -29)
  line L2033 (11, -23.3431) -> (11, -26.6569)
  line L2034 (10, -27.0711) -> (12.9289, -30)
  line L2035 (12.9289, -30) -> (17.0711, -30)
  line L2036 (17.0711, -30) -> (20, -27.0711)
  line L2037 (20, -27.0711) -> (20, -22.9289)
  line L2038 (20, -22.9289) -> (17.0711, -20)
  line L2039 (20, -22.9289) -> (20, -27.0711)
  line L2040 (22.9289, -20) -> (20, -22.9289)
  line L2041 (23.3431, -21) -> (21, -23.3431)
  line L2042 (26.6569, -21) -> (23.3431, -21)
  line L2043 (29, -23.3431) -> (26.6569, -21)
  line L2044 (29, -26.6569) -> (29, -23.3431)
  line L2045 (26.6569, -29) -> (29, -26.6569)
  line L2046 (23.3431, -29) -> (26.6569, -29)
  line L2047 (21, -26.6569) -> (23.3431, -29)
  line L2048 (21, -23.3431) -> (21, -26.6569)
  line L2049 (20, -27.0711) -> (22.9289, -30)
  line L2050 (22.9289, -30) -> (27.0711, -30)
  line L2051 (27.0711, -30) -> (30, -27.0711)
  line L2052 (30, -27.0711) -> (30, -22.9289)
  line L2053 (30, -22.9289) -> (27.0711, -20)
  line L2054 (30, -22.9289) -> (30, -27.0711)
  line L2055 (32.9289, -20) -> (30, -22.9289)
  line L2056 (33.3431, -21) -> (31, -23.3431)
  line L2057 (36.6569, -21) -> (33.3431, -21)
  line L2058 (39, -23.3431) -> (36.6569, -21)
  line L2059 (39, -26.6569) -> (39, -23.3431)
  line L2060 (36.6569, -29) -> (39, -26.6569)
  line L2061 (33.3431, -29) -> (36.6569, -29)
  line L2062 (31, -26.6569) -> (33.3431, -29)
  line L2063 (31, -23.3431) -> (31, -26.6569)
  line L2064 (30, -27.0711) -> (32.9289, -30)
  line L2065 (32.9289, -30) -> (37.0711, -30)
  line L2066 (37.0711, -30) -> (40, -27.0711)
  line L2067 (40, -27.0711) -> (40, -22.9289)
  line L2068 (40, -22.9289) -> (37.0711, -20)
  line L2069 (40, -22.9289) -> (40, -27.0711)
  line L2070 (42.9289, -20) -> (40, -22.9289)
  line L2071 (43.3431, -21) -> (41, -23.3431)
  line L2072 (46.6569, -21) -> (43.3431, -21)
  line L2073 (49, -23.3431) -> (46.6569, -21)
  line L2074 (49, -26.6569) -> (49, -23.3431)
  line L2075 (46.6569, -29) -> (49, -26.6569)
  line L2076 (43.3431, -29) -> (46.6569, -29)
  line L2077 (41, -26.6569) -> (43.3431, -29)
  line L2078 (41, -23.3431) -> (41, -26.6569)
  line L2079 (40, -27.0711) -> (42.9289, -30)
  line L2080 (42.9289, -30) -> (47.0711, -30)
  line L2081 (47.0711, -30) -> (50, -27.0711)
  line L2082 (50, -27.0711) -> (50, -22.9289)
  line L2083 (50, -22.9289) -> (47.0711, -20)
  line L2084 (50, -22.9289) -> (50, -27.0711)
  line L2085 (52.9289, -20) -> (50, -22.9289)
  line L2086 (53.3431, -21) -> (51, -23.3431)
  line L2087 (56.6569, -21) -> (53.3431, -21)
  line L2088 (59, -23.3431) -> (56.6569, -21)
  line L2089 (59, -26.6569) -> (59, -23.3431)
  line L2090 (56.6569, -29) -> (59, -26.6569)
  line L2091 (53.3431, -29) -> (56.6569, -29)
  line L2092 (51, -26.6569) -> (53.3431, -29)
  line L2093 (51, -23.3431) -> (51, -26.6569)
  line L2094 (50, -27.0711) -> (52.9289, -30)
  line L2095 (52.9289, -30) -> (57.0711, -30)
  line L2096 (57.0711, -30) -> (60, -27.0711)
  line L2097 (60, -27.0711) -> (60, -22.9289)
  line L2098 (60, -22.9289) -> (57.0711, -20)
  line L2099 (60, -22.9289) -> (60, -27.0711)
  line L2100 (62.9289, -20) -> (60, -22.9289)
  line L2101 (63.3431, -21) -> (61, -23.3431)
  line L2102 (66.6569, -21) -> (63.3431, -21)
  line L2103 (69, -23.3431) -> (66.6569, -21)
  line L2104 (69, -26.6569) -> (69, -23.3431)
  line L2105 (66.6569, -29) -> (69, -26.6569)
  line L2106 (63.3431, -29) -> (66.6569, -29)
  line L2107 (61, -26.6569) -> (63.3431, -29)
  line L2108 (61, -23.3431) -> (61, -26.6569)
  line L2109 (60, -27.0711) -> (62.9289, -30)
  line L2110 (62.9289, -30) -> (67.0711, -30)
  line L2111 (67.0711, -30) -> (70, -27.0711)
  line L2112 (70, -27.0711) -> (70, -22.9289)
  line L2113 (70, -22.9289) -> (67.0711, -20)
  line L2114 (-70, -32.9289) -> (-70, -37.0711)
  line L2115 (-67.0711, -30) -> (-70, -32.9289)
  line L2116 (-66.6569, -31) -> (-69, -33.3431)
  line L2117 (-63.3431, -31) -> (-66.6569, -31)
  line L2118 (-61, -33.3431) -> (-63.3431, -31)
  line L2119 (-61, -36.6569) -> (-61, -33.3431)
  line L2120 (-63.3431, -39) -> (-61, -36.6569)
  line L2121 (-66.6569, -39) -> (-63.3431, -39)
  line L2122 (-69, -36.6569) -> (-66.6569, -39)
  line L2123 (-69, -33.3431) -> (-69, -36.6569)
  line L2124 (-70, -37.0711) -> (-67.0711, -40)
  line L2125 (-67.0711, -40) -> (-62.9289, -40)
  line L2126 (-62.9289, -40) -> (-60, -37.0711)
  line L2127 (-60, -37.0711) -> (-60, -32.9289)
  line L2128 (-60, -32.9289) -> (-62.9289, -30)
  line L2129 (-60, -32.9289) -> (-60, -37.0711)
  line L2130 (-57.0711, -30) -> (-60, -32.9289)
  line L2131 (-56.6569, -31) -> (-59, -33.3431)
  line L2132 (-53.3431, -31) -> (-56.6569, -31)
  line L2133 (-51, -33.3431) -> (-53.3431, -31)
  line L2134 (-51, -36.6569) -> (-51, -33.3431)
  line L2135 (-53.3431, -39) -> (-51, -36.6569)
  line L2136 (-56.6569, -39) -> (-53.3431, -39)
  line L2137 (-59, -36.6569) -> (-56.6569, -39)
  line L2138 (-59, -33.3431) -> (-59, -36.6569)
  line L2139 (-60, -37.0711) -> (-57.0711, -40)
  line L2140 (-57.0711, -40) -> (-52.9289, -40)
  line L2141 (-52.9289, -40) -> (-50, -37.0711)
  line L2142 (-50, -37.0711) -> (-50, -32.9289)
  line L2143 (-50, -32.9289) -> (-52.9289, -30)
  line L2144 (-50, -32.9289) -> (-50, -37.0711)
  line L2145 (-47.0711, -30) -> (-50, -32.9289)
  line L2146 (-46.6569, -31) -> (-49, -33.3431)
  line L2147 (-43.3431, -31) -> (-46.6569, -31)
  line L2148 (-41, -33.3431) -> (-43.3431, -31)
  line L2149 (-41, -36.6569) -> (-41, -33.3431)
  line L2150 (-43.3431, -39) -> (-41, -36.6569)
  line L2151 (-46.6569, -39) -> (-43.3431, -39)
  line L2152 (-49, -36.6569) -> (-46.6569, -39)
  line L2153 (-49, -33.3431) -> (-49, -36.6569)
  line L2154 (-50, -37.0711) -> (-47.0711, -40)
  line L2155 (-47.0711, -40) -> (-42.9289, -40)
  line L2156 (-42.9289, -40) -> (-40, -37.0711)
  line L2157 (-40, -37.0711) -> (-40, -32.9289)
  line L2158 (-40, -32.9289) -> (-42.9289, -30)
  line L2159 (-40, -32.9289) -> (-40, -37.0711)
  line L2160 (-37.0711, -30) -> (-40, -32.9289)
  line L2161 (-36.6569, -31) -> (-39, -33.3431)
  line L2162 (-33.3431, -31) -> (-36.6569, -31)
  line L2163 (-31, -33.3431) -> (-33.3431, -31)
  line L2164 (-31, -36.6569) -> (-31, -33.3431)
  line L2165 (-33.3431, -39) -> (-31, -36.6569)
  line L2166 (-36.6569, -39) -> (-33.3431, -39)
  line L2167 (-39, -36.6569) -> (-36.6569, -39)
  line L2168 (-39, -33.3431) -> (-39, -36.6569)
  line L2169 (-40, -37.0711) -> (-37.0711, -40)
  line L2170 (-37.0711, -40) -> (-32.9289, -40)
  line L2171 (-32.9289, -40) -> (-30, -37.0711)
  line L2172 (-30, -37.0711) -> (-30, -32.9289)
  line L2173 (-30, -32.9289) -> (-32.9289, -30)
  line L2174 (-30, -32.9289) -> (-30, -37.0711)
  line L2175 (-27.0711, -30) -> (-30, -32.9289)
  line L2176 (-26.6569, -31) -> (-29, -33.3431)
  line L2177 (-23.3431, -31) -> (-26.6569, -31)
  line L2178 (-21, -33.3431) -> (-23.3431, -31)
  line L2179 (-21, -36.6569) -> (-21, -33.3431)
  line L2180 (-23.3431, -39) -> (-21, -36.6569)
  line L2181 (-26.6569, -39) -> (-23.3431, -39)
  line L2182 (-29, -36.6569) -> (-26.6569, -39)
  line L2183 (-29, -33.3431) -> (-29, -36.6569)
  line L2184 (-30, -37.0711) -> (-27.0711, -40)
  line L2185 (-27.0711, -40) -> (-22.9289, -40)
  line L2186 (-22.9289, -40) -> (-20, -37.0711)
  line L2187 (-20, -37.0711) -> (-20, -32.9289)
  line L2188 (-20, -32.9289) -> (-22.9289, -30)
  line L2189 (-20, -32.9289) -> (-20, -37.0711)
  line L2190 (-17.0711, -30) -> (-20, -32.9289)
  line L2191 (-16.6569, -31) -> (-19, -33.3431)
  line L2192 (-13.3431, -31) -> (-16.6569, -31)
  line L2193 (-11, -33.3431) -> (-13.3431, -31)
  line L2194 (-11, -36.6569) -> (-11, -33.3431)
  line L2195 (-13.3431, -39) -> (-11, -36.6569)
  line L2196 (-16.6569, -39) -> (-13.3431, -39)
  line L2197 (-19, -36.6569) -> (-16.6569, -39)
  line L2198 (-19, -33.3431) -> (-19, -36.6569)
  line L2199 (-20, -37.0711) -> (-17.0711, -40)
  line L2200 (-17.0711, -40) -> (-12.9289, -40)
  line L2201 (-12.9289, -40) -> (-10, -37.0711)
  line L2202 (-10, -37.0711) -> (-10, -32.9289)
  line L2203 (-10, -32.9289) -> (-12.9289, -30)
  line L2204 (-10, -32.9289) -> (-10, -37.0711)
  line L2205 (-7.0711, -30) -> (-10, -32.9289)
  line L2206 (-6.6569, -31) -> (-9, -33.3431)
  line L2207 (-3.3431, -31) -> (-6.6569, -31)
  line L2208 (-1, -33.3431) -> (-3.3431, -31)
  line L2209 (-1, -36.6569) -> (-1, -33.3431)
  line L2210 (-3.3431, -39) -> (-1, -36.6569)
  line L2211 (-6.6569, -39) -> (-3.3431, -39)
  line L2212 (-9, -36.6569) -> (-6.6569, -39)
  line L2213 (-9, -33.3431) -> (-9, -36.6569)
  line L2214 (-10, -37.0711) -> (-7.0711, -40)
  line L2215 (-7.0711, -40) -> (-2.9289, -40)
  line L2216 (-2.9289, -40) -> (0, -37.0711)
  line L2217 (0, -37.0711) -> (0, -32.9289)
  line L2218 (0, -32.9289) -> (-2.9289, -30)
  line L2219 (0, -32.9289) -> (0, -37.0711)
  line L2220 (2.9289, -30) -> (0, -32.9289)
  line L2221 (3.3431, -31) -> (1, -33.3431)
  line L2222 (6.6569, -31) -> (3.3431, -31)
  line L2223 (9, -33.3431) -> (6.6569, -31)
  line L2224 (9, -36.6569) -> (9, -33.3431)
  line L2225 (6.6569, -39) -> (9, -36.6569)
  line L2226 (3.3431, -39) -> (6.6569, -39)
  line L2227 (1, -36.6569) -> (3.3431, -39)
  line L2228 (1, -33.3431) -> (1, -36.6569)
  line L2229 (0, -37.0711) -> (2.9289, -40)
  line L2230 (2.9289, -40) -> (7.0711, -40)
  line L2231 (7.0711, -40) -> (10, -37.0711)
  line L2232 (10, -37.0711) -> (10, -32.9289)
  line L2233 (10, -32.9289) -> (7.0711, -30)
  line L2234 (10, -32.9289) -> (10, -37.0711)